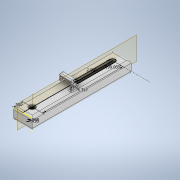
# Autodesk Inventor part: Elevator arm
Saved by Autodesk Inventor 2020 (Build 240168000, 168)
## iProperties
Created: 2022-01-06
Part Number: Elevator arm
Material: Generic
Document SubType Name: Modeling
Designer: pab2
Density: 1 g/cm^3
Appearance: Default
Author: pab2
Autodesk Inventor part; units mm, degrees
ref_plane "YZ Plane" through (0, 0, 0) normal (1, 0, 0) x (0, 1, 0)
ref_plane "XZ Plane" through (0, 0, 0) normal (0, 1, 0) x (-1, 0, 0)
ref_plane "XY Plane" through (0, 0, 0) normal (0, 0, 1) x (1, 0, 0)
sketch "Sketch1" plane through (0, 0, 0) normal (0, 1, 0) x (-1, 0, 0)
  line L0 (0, 0) -> (25.4, 0)
  line L1 (25.4, 0) -> (25.4, -136.0678)
  line L2 (25.4, -136.0678) -> (0, -136.0678)
  line L3 (0, -136.0678) -> (0, 0)
  dimension "d0" = 25.4
  dimension "d1" = 136.0678
  constraints: 8 end point, 2 parallel, 1 horizontal, 1 perpendicular
  measures "d0" distance of L1.end L2.end
  measures "d1" distance of L0.end L1.end
extrude "Extrusion1" add sketch "Sketch1" along normal blind 15.875
sketch "Sketch2" plane through (0, 15.875, 0) normal (0, 1, 0) x (1, 0, 0)
  line L0 (-25.4, 0) -> (0, 0) projected
  line L1 (-12.7, 0) -> (-12.7, 12.7)
  line L2 (-12.7, 12.7) -> (-12.7, 123.3678)
  line L3 (-12.7, 123.3678) -> (-12.7, 72.5678) construction
  line L4 (-16.002, 123.3678) -> (-16.002, 72.5678)
  line L5 (-9.398, 72.5678) -> (-9.398, 123.3678)
  arc A0 (-9.398, 123.3678) -> (-16.002, 123.3678) centre (-12.7, 123.3678) ccw
  arc A1 (-16.002, 72.5678) -> (-9.398, 72.5678) centre (-12.7, 72.5678) ccw
  line L6 (-12.7, 123.3678) -> (38.1, 123.3678) construction
  point P0 (-12.7, 97.9678)
  dimension "d4" = 12.7
  dimension "d5" = 110.6678
  dimension "d32" = 50.8
  dimension "d33" = 90
  dimension "d34" = 6.604
  constraints: 14 end point, 4 point on circle, 4 tangent, 2 centre point, 2 midpoint, 1 collinear, 1 horizontal, 1 parallel, 1 perpendicular, 1 point on line, 1 vertical
  measures "d4" distance of L1.start L1.end
  measures "d5" distance of L1.end L2.end
  measures "d32" distance of L2.end L3.end
  measures "d33" angle of L3 L6
  measures "d34" diameter of A1
hole "Hole1" at (-12.7, 15.875, -123.3678) direction (0, -1, 0) diameter 6.7564 end through all clearance for "Socket Head Cap Screw" size "1/4" standard "Ansi Unified Screw Threads"
fillet "Fillet1" radius 3.175 8 edges at (-25.4, 15.875, -68.0339) (0, 15.875, -68.0339) (-12.7, 15.875, 0) (-12.7, 0, 0) (-12.7, 15.875, -136.0678) (-12.7, 0, -136.0678) (0, 0, -68.0339) (-25.4, 0, -68.0339)
sketch "Sketch3" plane through (0, 15.875, 0) normal (0, 1, 0) x (1, 0, 0)
  line L0 (-22.225, 3.175) -> (-22.225, 132.8928) projected
  line L1 (-3.175, 3.175) -> (-22.225, 3.175) projected
  line L2 (-22.225, 132.8928) -> (-22.225, 3.175)
  line L3 (-22.225, 3.175) -> (-22.225, 61.6839)
  line L4 (-22.225, 61.6839) -> (-22.225, 58.5089)
  line L5 (-22.225, 58.5089) -> (-3.175, 58.5089)
  line L6 (-3.175, 132.8928) -> (-3.175, 3.175) projected
  line L7 (-3.175, 58.5089) -> (-3.175, 64.8589)
  line L8 (-22.225, 58.5089) -> (-3.175, 58.5089)
  line L9 (-3.175, 58.5089) -> (-3.175, 64.8589)
  line L10 (-3.175, 64.8589) -> (-22.225, 64.8589)
  line L11 (-22.225, 64.8589) -> (-22.225, 58.5089)
  point P0 (0, 0)
  dimension "d14" = 58.5089
  dimension "d15" = 0
  dimension "d16" = 3.175
  dimension "d17" = 6.35
  constraints: 18 end point, 3 point on line, 2 parallel, 2 perpendicular, 1 collinear, 1 horizontal, 1 vertical
  measures "d14" distance of L0.start L3.end
  measures "d15" distance between parallel lines of L3 L2
  measures "d16" distance of L3.end L4.end
  measures "d17" distance of L5.end L7.end
extrude "Extrusion2" add sketch "Sketch3" along normal blind 12.7 contours L0 L10 L6 L5
sketch "Sketch4" plane through (-22.225, 15.875, -58.5089) normal (0, 0, 1) x (1, 0, 0)
  line L0 (19.05, 12.7) -> (0, 12.7)
  line L1 (19.05, 12.7) -> (15.457898, 9.107898)
  line L2 (19.05, 12.7) -> (24.13, 12.7) construction
  line L3 (19.05, 0) -> (0, 0)
  line L4 (15.457898, 9.107898) -> (3.885116, 9.107898)
  line L5 (3.885116, 9.107898) -> (3.885116, 0)
  line L6 (3.885116, 0) -> (15.457898, 0)
  line L7 (15.457898, 0) -> (15.457898, 9.107898)
  line L8 (0, 0) -> (0, 12.7)
  line L9 (3.885116, 0) -> (0, 0)
  line L10 (0, 0) -> (0, 5.004372)
  line L11 (0, 5.004372) -> (3.885116, 5.004372)
  line L12 (3.885116, 5.004372) -> (3.885116, 0)
  point P0 (22.225, -15.875)
  point P1 (3.885116, 5.004372)
  dimension "d20" = 5.08
  dimension "d21" = 135
  constraints: 20 end point, 4 parallel, 3 horizontal, 2 perpendicular, 2 point on line, 1 equal length
  measures "d20" distance of L0.start L1.end
  measures "d21" angle of L1 L2
extrude "Extrusion3" cut sketch "Sketch4" against normal blind 12.7 contours L7 L3 L5 L4 | L11 L5 L3 L8
fillet "Fillet2" radius 1.5875 19 edges at (-3.175, 22.225, -58.5089) (-6.7671, 20.4289, -58.5089) (-12.5535, 24.9829, -58.5089) (-12.7, 28.575, -58.5089) (-3.175, 28.575, -61.6839) (-3.175, 22.225, -64.8589) (-3.175, 15.875, -61.6839) (-12.7, 28.575, -64.8589) (-22.225, 28.575, -61.6839) (-18.3399, 22.9311, -58.5089) (-22.225, 24.7272, -58.5089) (-18.3399, 20.8794, -61.6839) (-22.225, 24.7272, -64.8589) (-18.3399, 22.9311, -64.8589) (-12.5535, 24.9829, -64.8589) (-6.7671, 20.4289, -64.8589) (-4.9711, 15.875, -64.8589) (-6.7671, 15.875, -61.6839) (-4.9711, 15.875, -58.5089)
hole "Hole2" at (-12.7, 15.875, -12.7) direction (0, -1, 0) diameter 8.4328 end through all clearance for "Socket Head Cap Screw" size "5/16" standard "Ansi Unified Screw Threads"
extrude "Extrusion4" cut sketch "Sketch2" against normal through all
sketch "Sketch6" plane through (0, 0, 0) normal (0, -1, 0) x (1, 0, 0)
  circle A0 centre (-12.7, -12.7) radius 4.2164 projected
  circle A1 centre (-12.7, -12.7) radius 5.461
  circle A2 centre (-12.7, -12.7) radius 6.35
  point P0 (0, 0)
  dimension "d39" = 10.922
  dimension "d40" = 12.7
  constraints: 2 centre point, 2 coincident
  measures "d39" diameter of A1
  measures "d40" diameter of A2
extrude "Extrusion5" cut sketch "Sketch6" against normal blind 12.7 contours A1
ref_plane "Work Plane1" through (-12.7, 0, -12.7) normal (1, 0, 0) x (0, 0, -1)
sketch "Sketch8" plane through (-12.7, 0, -12.7) normal (1, 0, 0) x (0, 0, -1)
  line L0 (5.461, 0) -> (-5.461, 0)
  line L1 (0, 0) -> (6.35, 0)
  line L2 (0, 0) -> (6.35, 0) construction
  line L3 (6.35, 0) -> (5.461, 12.713522)
  line L4 (5.461, 12.713522) -> (5.461, 0)
  line L5 (5.461, 0) -> (5.461, 12.7)
  line L6 (0, 34.29) -> (0, -5.715)
  point P0 (-12.7, 0)
  dimension "d48" = 6.35
  dimension "d49" = 0
  constraints: 8 end point, 2 collinear, 2 point on line, 1 horizontal, 1 midpoint
  measures "d48" distance of L1.start L1.end
  measures "d49" distance between parallel lines of L1 L2
sketch "Sketch8 outline for Revolution1" plane through (-12.7, 0, -12.7) normal (1, 0, 0) x (0, 0, -1)
  line L0 (6.35, 0) -> (5.461, 12.713522)
  line L1 (5.461, 0) -> (6.35, 0)
  line L2 (5.461, 12.713522) -> (5.461, 0)
revolve "Revolution1" cut sketch "Sketch8 outline for Revolution1" angle 360 about axis through (-12.7, 15.875, -12.7) along (0, -1, 0)
body "Solid1"
